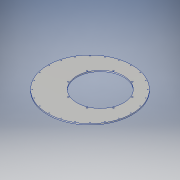
# Autodesk Inventor part: 55K stage
Saved by Autodesk Inventor 2018 (Build 220112000, 112)
## iProperties
Created: 2018-10-14
Part Number: 55K stage
Material: Aluminum 6061
Document SubType Name: Modeling
Designer: freyja
Density: 2.7 g/cm^3
Appearance: Aluminum - Flat
Mass: 2661.5 g
Surface Area: 3217.19 cm^2
Volume: 985.742 cm^3
Author: freyja
Autodesk Inventor part; units mm, degrees
note: some values were not read from the file. Chosen so that the rebuilt part matches the saved one: direction of "Hole3".
ref_plane "YZ Plane" through (0, 0, 0) normal (1, 0, 0) x (0, 1, 0)
ref_plane "XZ Plane" through (0, 0, 0) normal (0, 1, 0) x (-1, 0, 0)
ref_plane "XY Plane" through (0, 0, 0) normal (0, 0, 1) x (1, 0, 0)
sketch "Sketch1" plane through (0, 0, 0) normal (0, 1, 0) x (-1, 0, 0)
  circle A0 centre (0, 0) radius 228.6
  dimension "d0" = 457.2
  constraints: 1 centre point, 1 coincident
  measures "d0" diameter of A0
extrude "Extrusion1" add sketch "Sketch1" along normal blind 6.35
sketch "Sketch7" plane through (0, 6.35, 0) normal (0, 1, 0) x (1, 0, 0)
  line L0 (0, 0) -> (0, 222.25)
  dimension "d42" = 222.25
  constraints: 2 end point, 1 vertical
  measures "d42" distance of L0.start L0.end
hole "Hole3" at (0, 6.35, -222.25) direction (0, -1, 0) diameter 3.302 end up to surface thread size "8-32 UNC" class "2B" standard "ANSI Unified Screw Threads"
pattern_circular "Circular Pattern1" count 24 over 360 about axis through (0, 0, 0) along (0, 1, 0) of "Hole3"
sketch "Sketch8" plane through (0, 6.35, 0) normal (0, 1, 0) x (1, 0, 0)
  line L0 (0, 0) -> (28.0184, 28.0184) construction
  line L1 (0, 0) -> (39.624, 0) construction
  circle A0 centre (28.0184, 28.0184) radius 127
  dimension "d53" = 39.624
  dimension "d54" = 45
  dimension "d55" = 254
  constraints: 4 end point, 1 centre point, 1 coincident, 1 equal length, 1 horizontal
  measures "d53" distance of L0.start L0.end
  measures "d54" angle of L1 L0
  measures "d55" diameter of A0
extrude "Extrusion4" cut sketch "Sketch8" against normal through all
sketch "Sketch9" plane through (0, 6.35, 0) normal (0, 1, 0) x (1, 0, 0)
  circle A0 centre (28.0184, 28.0184) radius 127 projected
  line L0 (28.0184, 28.0184) -> (151.2177, 79.0492)
  line L1 (28.0184, 28.0184) -> (161.3684, 28.0184) construction
  point P0 (0, 0)
  dimension "d58" = 133.35
  dimension "d59" = 22.5
  constraints: 4 end point, 1 equal length, 1 horizontal
  measures "d58" distance of L0.start L0.end
  measures "d59" angle of L1 L0
hole "Hole4" at (151.2177, 6.35, -79.0492) direction (0, -1, 0) diameter 6.7564 end through all clearance for "Flat Head Machine Screw (82)" size "1/4" standard "Ansi Unified Screw Threads"
pattern_circular "Circular Pattern2" count 8 over 360 about axis through (28.0184, 6.35, -28.0184) along (0, -1, 0) of "Hole4"
body "Solid1"
